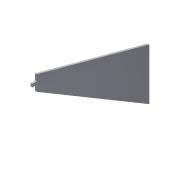
# Autodesk Inventor part: ControlRightPanel
Saved by Autodesk Inventor 2014 (Build 180170000, 170)
## iProperties
Created: 2015-01-19
Part Number: ControlRightPanel
Material: Generic
Document SubType Name: Modeling
Designer: Peele
Density: 1 g/cm^3
Appearance: White
Author: Peele
Autodesk Inventor part; units mm, degrees
ref_plane "YZ Plane" through (0, 0, 0) normal (1, 0, 0) x (0, 1, 0)
ref_plane "XZ Plane" through (0, 0, 0) normal (0, 1, 0) x (-1, 0, 0)
ref_plane "XY Plane" through (0, 0, 0) normal (0, 0, 1) x (1, 0, 0)
sketch "Sketch1" plane through (0, 0, 0) normal (1, 0, 0) x (0, 1, 0)
  line L0 (0, 0) -> (0, 25)
  line L1 (0, 25) -> (185, -25)
  line L2 (185, -25) -> (185, -110)
  line L3 (185, -110) -> (0, 0)
  dimension "d0" = 25
  dimension "d1" = 85
  dimension "d2" = 185
  dimension "d10" = 25
  constraints: 8 end point, 1 parallel, 1 vertical
  measures "d0" distance of L0.start L0.end
  measures "d1" distance of L1.end L2.end
  measures "d2" distance between parallel lines of L0 L2
  measures "d10" vertical distance of L0.start L1.end
extrude "Extrusion1" add sketch "Sketch1" along normal blind 3
sketch "Sketch2" plane through (3, 0, 0) normal (1, 0, 0) x (0, 0, -1)
  line L0 (-25, 0) -> (0, 0) projected
  line L1 (-15, 0) -> (-10, 0)
  line L2 (-10, 0) -> (-10, -7.5)
  line L3 (-10, -7.5) -> (-15, -7.5)
  line L4 (-15, -7.5) -> (-15, 0)
  dimension "d5" = 5
  dimension "d6" = 7.5
  dimension "d7" = 10
  constraints: 8 end point, 2 parallel, 1 horizontal, 1 perpendicular, 1 point on line
  measures "d5" distance of L2.end L3.end
  measures "d6" distance from line of L0.end L3
  measures "d7" distance from line of L0.end L2
extrude "Extrusion2" add sketch "Sketch2" against normal blind 3
body "Solid1"
